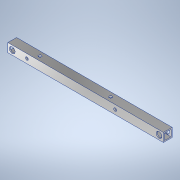
# Autodesk Inventor part: ロボット回転9x9_3
Saved by Autodesk Inventor 2020.3 (Build 243373000, 373)
## iProperties
Created: 2020-07-05
Part Number: ロボット回転9x9_3
Material: アルミニウム 6061
Document SubType Name: Modeling
Designer: totot
Density: 2.7 g/cm^3
Appearance: アルミニウム - フラット
Mass: 12.5422 g
Surface Area: 79.9795 cm^2
Volume: 4.64527 cm^3
Author: totot
Autodesk Inventor part; units mm, degrees
ref_plane "YZ Plane" through (0, 0, 0) normal (1, 0, 0) x (0, 1, 0)
ref_plane "XZ Plane" through (0, 0, 0) normal (0, 1, 0) x (-1, 0, 0)
ref_plane "XY Plane" through (0, 0, 0) normal (0, 0, 1) x (1, 0, 0)
sketch "スケッチ1" plane through (0, 0, 0) normal (1, 0, 0) x (0, 1, 0)
  line L0 (0, 0) -> (9, 0)
  line L1 (9, 0) -> (9, 9)
  line L2 (9, 9) -> (0, 9)
  line L3 (0, 9) -> (0, 0)
  line L4 (1.2, 7.8) -> (7.8, 7.8)
  line L5 (7.8, 7.8) -> (7.8, 1.2)
  line L6 (7.8, 1.2) -> (1.2, 1.2)
  line L7 (1.2, 1.2) -> (1.2, 7.8)
  dimension "d0" = 9
  dimension "d1" = 9
  dimension "d2" = 6.6
  dimension "d3" = 6.6
  dimension "d4" = 1.2
  dimension "d5" = 1.2
  constraints: 16 end point, 4 parallel, 2 horizontal, 2 perpendicular
  measures "d0" distance of L2.end L1.end
  measures "d1" distance of L1.end L0.end
  measures "d2" distance of L5.end L6.end
  measures "d3" distance of L6.end L4.start
  measures "d4" distance between parallel lines of L0 L6
  measures "d5" distance between parallel lines of L7 L3
extrude "押し出し1" add sketch "スケッチ1" along normal blind 99.5097
sketch "スケッチ2" plane through (0, 0, 9) normal (0, 0, 1) x (1, 0, 0)
  line L0 (0, 9) -> (0, 0) projected
  line L1 (0, 9) -> (99.5097, 9) projected
  line L2 (99.5097, 9) -> (99.5097, 0) projected
  point P0 (4.5, 4.5)
  point P1 (95.0097, 4.5)
  dimension "d8" = 4.5
  dimension "d9" = 4.5
  dimension "d10" = 4.5
  dimension "d11" = 4.5
  measures "d8" distance from line of point (4.5, 4.5) L0
  measures "d9" distance from line of point (4.5, 4.5) L1
  measures "d10" distance from line of L2 point (95.01, 4.5)
  measures "d11" distance from line of L1 point (95.01, 4.5)
hole "穴1" at (4.5, 4.5, 9) at (95.0097, 4.5, 9) direction (0, 0, -1) diameter 3 end through all
sketch "スケッチ3" plane through (0, 9, 9) normal (0, 1, 0) x (1, 0, 0)
  line L0 (0, 0) -> (99.5097, 0) projected
  line L1 (0, 9) -> (0, 0) projected
  line L2 (99.5097, 9) -> (99.5097, 0) projected
  point P0 (13.5, 4.5)
  point P1 (86.0097, 4.5)
  dimension "d19" = 4.5
  dimension "d20" = 13.5
  dimension "d21" = 13.5
  dimension "d22" = 4.5
  measures "d19" distance from line of point (13.5, 4.5) L0
  measures "d20" distance from line of point (13.5, 4.5) L1
  measures "d21" distance from line of L2 point (86.01, 4.5)
  measures "d22" distance from line of L0 point (86.01, 4.5)
hole "穴2" at (13.5, 9, 4.5) at (86.0097, 9, 4.5) direction (0, -1, 0) diameter 3 end through all
sketch "スケッチ4" plane through (99.5097, 0, 0) normal (1, 0, 0) x (0, 0, -1)
  line L0 (0, 9) -> (-9, 9) projected
  line L1 (0, 0) -> (-9, 0)
  line L2 (-9, 0) -> (-9, 9)
  line L3 (-9, 9) -> (0, 9)
  line L4 (0, 9) -> (0, 0)
  line L5 (-1.2, 1.2) -> (-7.8, 1.2) projected
  line L6 (-7.8, 1.2) -> (-7.8, 7.8) projected
  line L7 (-1.2, 1.2) -> (-7.8, 1.2)
  line L8 (-7.8, 1.2) -> (-7.8, 7.8)
  line L9 (-7.8, 7.8) -> (-1.2, 7.8)
  line L10 (-1.2, 7.8) -> (-1.2, 1.2)
  dimension "d30" = 6.6
  dimension "d31" = 6.6
  constraints: 16 end point, 4 parallel, 2 horizontal, 2 perpendicular
  measures "d30" distance of L6.end L9.end
  measures "d31" distance of L7.end L6.end
extrude "押し出し2" add sketch "スケッチ4" along normal blind 55
sketch "スケッチ5" plane through (0, 0, 0) normal (-1, 0, 0) x (0, 0, 1)
  line L0 (0, 9) -> (9, 9) projected
  line L1 (0, 0) -> (9, 0)
  line L2 (9, 0) -> (9, 9)
  line L3 (9, 9) -> (0, 9)
  line L4 (0, 9) -> (0, 0)
  line L5 (1.2, 1.2) -> (7.8, 1.2) projected
  line L6 (7.8, 1.2) -> (7.8, 7.8) projected
  line L7 (1.2, 1.2) -> (7.8, 1.2)
  line L8 (7.8, 1.2) -> (7.8, 7.8)
  line L9 (7.8, 7.8) -> (1.2, 7.8)
  line L10 (1.2, 7.8) -> (1.2, 1.2)
  constraints: 16 end point, 4 parallel, 2 horizontal, 2 perpendicular
extrude "押し出し3" add sketch "スケッチ5" along normal blind 15
sketch "スケッチ6" plane through (154.5097, 0, 0) normal (0, 0, -1) x (-1, 0, 0)
  line L0 (169.5097, 9) -> (169.5097, 0) projected
  line L1 (0, 9) -> (169.5097, 9) projected
  line L2 (0, 0) -> (0, 9) projected
  point P0 (154.5097, 0)
  point P1 (165.0097, 4.5)
  point P2 (4.5, 4.5)
  dimension "d36" = 4.5
  dimension "d37" = 4.5
  dimension "d38" = 4.5
  dimension "d39" = 4.5
  measures "d36" distance from line of point (165.01, 4.5) L0
  measures "d37" distance from line of point (165.01, 4.5) L1
  measures "d38" distance from line of L1 point (4.5, 4.5)
  measures "d39" distance from line of point (4.5, 4.5) L2
hole "穴3" at (-10.5, 4.5, 0) at (150.0097, 4.5, 0) direction (0, 0, 1) diameter 6 end through all
sketch "スケッチ7" plane through (154.5097, 9, 9) normal (0, 1, 0) x (1, 0, 0)
  line L0 (0, 9) -> (0, 0) projected
  circle A0 centre (-68.5, 4.5) radius 1.5 projected
  line L1 (0, 9) -> (-169.5097, 9) projected
  point P0 (-154.5097, 9)
  point P1 (-53.5, 4.5)
  point P2 (-20, 4.5)
  dimension "d47" = 20
  dimension "d48" = 15
  dimension "d49" = 4.5
  dimension "d50" = 4.5
  measures "d47" distance from line of point (-20, 4.5) L0
  measures "d48" distance of point (-53.5, 4.5) A0.centre
  measures "d49" distance from line of point (-53.5, 4.5) L1
  measures "d50" distance from line of point (-20, 4.5) L1
hole "穴4" at (101.0097, 9, 4.5) at (134.5097, 9, 4.5) direction (0, -1, 0) diameter 3 end through all
equation "\"d3\" = d2"
equation "\"d5\" = d4"
equation "\"d9\" = d8"
equation "\"d37\" = d36"
equation "\"d38\" = d36"
equation "\"d39\" = d38"
equation "\"d50\" = d49"
